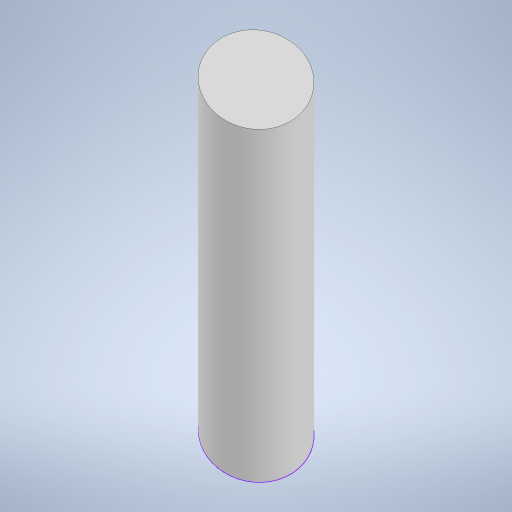
# Autodesk Inventor part: REMEDIO5
Saved by Autodesk Inventor 2023 (Build 270158000, 158)
## iProperties
Created: 2023-03-02
Part Number: REMEDIO5
Material: Generic
Document SubType Name: Modeling
Designer: accam
Density: 1 g/cm^3
Appearance: Default
Author: accam
Autodesk Inventor part; units mm, degrees
ref_plane "YZ Plane" through (0, 0, 0) normal (1, 0, 0) x (0, 1, 0)
ref_plane "XZ Plane" through (0, 0, 0) normal (0, 1, 0) x (-1, 0, 0)
ref_plane "XY Plane" through (0, 0, 0) normal (0, 0, 1) x (1, 0, 0)
sketch "Sketch2" plane through (0, 0, 0) normal (0, 1, 0) x (-1, 0, 0)
  ellipse E0 centre (0.0124, 0.0552) end of major axis (-7.53, 6.6212) minor radius 6.6814
  point P0 (0, 0)
  point P1 (0, 0)
  constraints: 1 coincident, 2 other
extrude "Extrusion1" add sketch "Sketch2" along normal blind 50
body "Solid1"
